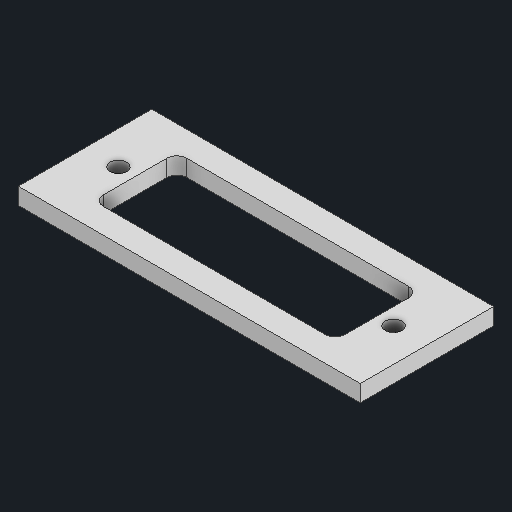
# Autodesk Inventor part: DMF 01 54 lower sheet v2.1
Saved by Autodesk Inventor 2026.2 (Build 302298010, 298A)
## iProperties
Created: 2024-05-05
Part Number: DMF 01 54 lower sheet v2.1
Material: Generic
Document SubType Name: Modeling
Designer: pokla
Density: 1 g/cm^3
Appearance: Default
Author: pokla
Autodesk Inventor part; units mm, degrees
ref_plane "YZ Plane" through (0, 0, 0) normal (1, 0, 0) x (0, 1, 0)
ref_plane "XZ Plane" through (0, 0, 0) normal (0, 1, 0) x (-1, 0, 0)
ref_plane "XY Plane" through (0, 0, 0) normal (0, 0, 1) x (1, 0, 0)
sketch "Sketch4" plane through (0, 0, 0) normal (0, 1, 0) x (-1, 0, 0)
  line L0 (72.5, -25) -> (-72.5, -25)
  line L1 (-72.5, -25) -> (-72.5, 25)
  line L2 (-72.5, 25) -> (72.5, 25)
  line L3 (72.5, 25) -> (72.5, -25)
  line L4 (72.5, -25) -> (-72.5, 25) construction
  line L5 (-72.5, -25) -> (72.5, 25) construction
  line L6 (102.5, -40) -> (-102.5, -40)
  line L7 (-102.5, -40) -> (-102.5, 40)
  line L8 (-102.5, 40) -> (102.5, 40)
  line L9 (102.5, 40) -> (102.5, -40)
  line L10 (102.5, -40) -> (-102.5, 40) construction
  line L11 (-102.5, -40) -> (102.5, 40) construction
  circle A0 centre (82.5, 0) radius 5
  circle A1 centre (-82.5, 0) radius 5
  line L12 (0, -25) -> (0, 25) construction
  point P0 (0, 0)
  dimension "d23" = 145
  dimension "d24" = 50
  dimension "d25" = 205
  dimension "d26" = 80
  dimension "d27" = 165
  dimension "d28" = 10
  constraints: 26 end point, 6 midpoint, 4 parallel, 2 centre point, 2 horizontal, 2 horizontal alignment, 2 perpendicular, 1 other
  measures "d23" distance of L0.start L0.end
  measures "d24" distance of L0.end L1.end
  measures "d25" distance of L6.start L6.end
  measures "d26" distance of L6.end L7.end
  measures "d27" distance of A1.centre A0.centre
  measures "d28" diameter of A0
extrude "Extrusion3" add sketch "Sketch4" along normal blind 10
fillet "Fillet2" radius 6 4 edges at (-72.5, 5, -25) (72.5, 5, -25) (72.5, 5, 25) (-72.5, 5, 25)
body "Solid2"
